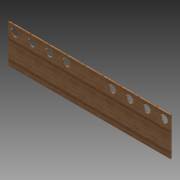
# Autodesk Inventor part: manipulator back pannel 2
Saved by Autodesk Inventor 2012 (Build 160160000, 160)
## iProperties
Created: 2013-09-02
Part Number: manipulator back pannel 2
Material: Default
Document SubType Name: Modeling
Designer: Bryce
Density: 1 g/cm^3
Author: Bryce
Autodesk Inventor part; units mm, degrees
ref_plane "YZ Plane" through (0, 0, 0) normal (1, 0, 0) x (0, 1, 0)
ref_plane "XZ Plane" through (0, 0, 0) normal (0, 1, 0) x (-1, 0, 0)
ref_plane "XY Plane" through (0, 0, 0) normal (0, 0, 1) x (1, 0, 0)
sketch "Sketch1" plane through (0, 0, 0) normal (0, 0, 1) x (1, 0, 0)
  line L0 (0, 0) -> (812.8, 0)
  line L1 (812.8, 0) -> (812.8, 190.5)
  line L2 (812.8, 190.5) -> (0, 190.5)
  line L3 (0, 190.5) -> (0, 0)
  circle A0 centre (781.05, 158.75) radius 19.05
  circle A1 centre (520.7, 158.75) radius 19.05
  circle A2 centre (292.1, 158.75) radius 19.05
  circle A3 centre (31.75, 158.75) radius 19.05
  circle A4 centre (694.2667, 158.75) radius 19.05
  circle A5 centre (205.3167, 158.75) radius 19.05
  circle A6 centre (607.4833, 158.75) radius 19.05
  circle A7 centre (118.5333, 158.75) radius 19.05
  dimension "d0" = 190.5
  dimension "d1" = 812.8
  dimension "d13" = 38.1
  dimension "d14" = 38.1
  dimension "d15" = 228.6
  dimension "d16" = 260.35
  dimension "d17" = 86.7833
  dimension "d18" = 86.7833
  dimension "d21" = 31.75
  dimension "d22" = 31.75
  dimension "d23" = 31.75
  dimension "d24" = 86.7833
  dimension "d25" = 86.7833
  constraints: 8 centre point, 8 end point, 7 horizontal alignment, 6 equal radius, 2 parallel, 1 coincident, 1 horizontal, 1 perpendicular
  measures "d0" distance of L2.end L0.start
  measures "d1" distance of L1.end L2.end
  measures "d13" diameter of A0
  measures "d14" diameter of A1
  measures "d15" distance of A2.centre A1.centre
  measures "d16" distance of A1.centre A0.centre
  measures "d17" distance of A4.centre A0.centre
  measures "d18" distance of A5.centre A2.centre
  measures "d21" distance from line of L2 A3.centre
  measures "d22" distance from line of L3 A3.centre
  measures "d23" distance from line of L1 A0.centre
  measures "d24" distance of A6.centre A4.centre
  measures "d25" distance of A7.centre A5.centre
extrude "Extrusion1" add sketch "Sketch1" along normal blind 6.35
equation "\"d14\" = d13"
equation "\"d16\" = 0.5 * d1 - 0.5 * d15 - d23"
equation "\"d17\" = 0.333333 * d16"
equation "\"d18\" = d17"
equation "\"d23\" = d22"
equation "\"d24\" = d17"
equation "\"d25\" = d18"
body "Solid1"
